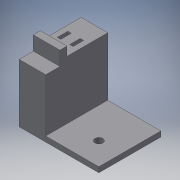
# Autodesk Inventor part: FixedFiber
Saved by Autodesk Inventor 2019 (Build 230136000, 136)
## iProperties
Created: 2019-06-10
Part Number: FixedFiber
Material: Generic
Document SubType Name: Modeling
Designer: aorfi
Density: 1 g/cm^3
Appearance: Default
Author: aorfi
Autodesk Inventor part; units mm, degrees
ref_plane "YZ Plane" through (0, 0, 0) normal (1, 0, 0) x (0, 1, 0)
ref_plane "XZ Plane" through (0, 0, 0) normal (0, 1, 0) x (-1, 0, 0)
ref_plane "XY Plane" through (0, 0, 0) normal (0, 0, 1) x (1, 0, 0)
sketch "Sketch1" plane through (0, 0, 0) normal (0, 1, 0) x (-1, 0, 0)
  line L0 (-22.5, 17.5) -> (22.5, 17.5)
  line L1 (22.5, 17.5) -> (22.5, -17.5)
  line L2 (22.5, -17.5) -> (-22.5, -17.5)
  line L3 (-22.5, -17.5) -> (-22.5, 17.5)
  line L4 (-22.5, 17.5) -> (22.5, -17.5) construction
  line L5 (22.5, 17.5) -> (-22.5, -17.5) construction
  point P0 (0, 0)
  dimension "d0" = 35
  dimension "d1" = 45
  constraints: 12 end point, 2 midpoint, 2 parallel, 1 horizontal, 1 perpendicular
  measures "d0" distance of L0.end L1.end
  measures "d1" distance of L1.end L2.end
extrude "Extrusion1" add sketch "Sketch1" along normal mid plane 3
sketch "Sketch2" plane through (0, 1.5, 0) normal (0, 1, 0) x (1, 0, 0)
  line L0 (-22.5, -17.5) -> (22.5, -17.5) projected
  line L1 (22.5, -17.5) -> (22.5, 17.5) projected
  point P0 (9.8, -4.8)
  dimension "d11" = 12.7
  dimension "d12" = 12.7
  measures "d11" distance from line of L0 point (9.8, -4.8)
  measures "d12" distance from line of L1 point (9.8, -4.8)
hole "Hole1" at (9.8, 1.5, 4.8) direction (0, -1, 0) diameter 4.496 end through all clearance for "Flat Head Machine Screw (82)" size "#8" standard "Ansi Unified Screw Threads"
sketch "Sketch3" plane through (0, 1.5, 0) normal (0, 1, 0) x (1, 0, 0)
  line L0 (22.5, 17.5) -> (-22.5, 17.5) projected
  line L1 (-22.5, 17.5) -> (-7.5, 17.5)
  line L2 (-7.5, 17.5) -> (-7.5, -17.5)
  line L3 (-7.5, -17.5) -> (-22.5, -17.5)
  line L4 (-22.5, -17.5) -> (-22.5, 17.5)
  line L5 (-22.5, -17.5) -> (22.5, -17.5) projected
  point P0 (0, 0)
  dimension "d13" = 15
  constraints: 8 end point, 2 parallel, 1 collinear, 1 horizontal, 1 perpendicular
  measures "d13" distance of L2.end L3.end
extrude "Extrusion2" add sketch "Sketch3" along normal blind 33
sketch "Sketch4" plane through (0, 34.5, 0) normal (0, 1, 0) x (1, 0, 0)
  line L0 (-7.5, -17.5) -> (-7.5, 17.5) projected
  line L1 (-22.5, -3.5) -> (-7.5, -3.5)
  line L2 (-7.5, -3.5) -> (-7.5, -7.5)
  line L3 (-7.5, -7.5) -> (-22.5, -7.5)
  line L4 (-22.5, -7.5) -> (-22.5, -3.5)
  line L5 (-22.5, 17.5) -> (-22.5, -17.5) projected
  line L6 (-22.5, -3.5) -> (-7.5, -3.5) construction
  line L7 (-7.5, -3.5) -> (-7.5, 3.5) construction
  line L8 (-7.5, 3.5) -> (-22.5, 3.5) construction
  line L9 (-22.5, 3.5) -> (-22.5, -3.5) construction
  line L10 (-22.5, -17.5) -> (-22.5, 17.5) construction
  line L11 (-22.5, 0) -> (-7.5, 0) construction
  line L12 (-22.5, -17.5) -> (-7.5, -17.5) projected
  point P0 (0, 0)
  dimension "d16" = 4
  dimension "d32" = 10
  constraints: 18 end point, 4 parallel, 4 point on line, 3 horizontal, 2 collinear, 2 midpoint, 2 perpendicular
  measures "d16" distance between parallel lines of L3 L1
  measures "d32" distance between parallel lines of L12 L3
extrude "Extrusion3" add sketch "Sketch4" along normal blind 5 contours L3 L4 L1 L0
sketch "Sketch5" plane through (0, 34.5, 0) normal (0, 1, 0) x (1, 0, 0)
  line L0 (-19.5, 9) -> (-17.5, 9)
  line L1 (-17.5, 9) -> (-17.5, 3)
  line L2 (-17.5, 3) -> (-19.5, 3)
  line L3 (-19.5, 3) -> (-19.5, 9)
  line L4 (-10.5, 9) -> (-12.5, 9)
  line L5 (-12.5, 9) -> (-12.5, 3)
  line L6 (-12.5, 3) -> (-10.5, 3)
  line L7 (-10.5, 3) -> (-10.5, 9)
  line L8 (-18.5, 6) -> (-11.5, 6) construction
  line L9 (-7.5, -3.5) -> (-22.5, -3.5) construction
  line L10 (-7.5, 11.5) -> (-7.5, 1.5) construction
  line L11 (-7.5, 1.5) -> (-22.5, 1.5) construction
  line L12 (-22.5, 17.5) -> (-22.5, -3.5) construction
  line L13 (-22.5, -17.5) -> (-22.5, 17.5) construction
  point P0 (0, 0)
  point P1 (-15, -3.5)
  point P2 (-15, 6)
  point P3 (-11.5, 9)
  point P4 (-18.5, 9)
  point P5 (-17.5, 6)
  dimension "d20" = 6
  dimension "d21" = 2
  dimension "d22" = 5
  dimension "d26" = 1.5
  dimension "d31" = 7
  constraints: 22 end point, 5 midpoint, 4 parallel, 3 horizontal, 3 point on line, 3 vertical alignment, 2 perpendicular, 1 collinear
  measures "d20" distance of L2.end L0.start
  measures "d21" distance of L0.start L0.end
  measures "d22" distance between parallel lines of L9 L11
  measures "d26" distance between parallel lines of L2 L11
  measures "d31" distance of L8.start L8.end
extrude "Extrusion4" cut sketch "Sketch5" against normal blind 3
sketch "Sketch7" plane through (-22.5, -1.5, -17.5) normal (-1, 0, 0) x (0, 0, 1)
  line L0 (35, 36) -> (25, 36)
  line L1 (25, 36) -> (25, 33)
  line L2 (25, 33) -> (35, 33)
  line L3 (35, 33) -> (35, 36)
  line L4 (25, 36) -> (25, 41) projected
  point P0 (17.5, 1.5)
  dimension "d33" = 3
  constraints: 8 end point, 2 parallel, 1 collinear, 1 horizontal, 1 perpendicular
  measures "d33" distance between parallel lines of L2 L0
extrude "Extrusion6" cut sketch "Sketch7" against normal through all
sketch "Sketch8" plane through (0, 34.5, 0) normal (0, 1, 0) x (1, 0, 0)
  line L0 (-22.5, -3.5) -> (-7.5, -3.5) projected
  line L1 (-7.5, -3.5) -> (-8.5, -3.5)
  line L2 (-8.5, -3.5) -> (-8.5, -1.5)
  line L3 (-8.5, -1.5) -> (-7.5, -1.5)
  line L4 (-7.5, -1.5) -> (-7.5, -3.5)
  point P0 (0, 0)
  dimension "d36" = 1
  dimension "d37" = 2
  constraints: 8 end point, 2 parallel, 1 horizontal, 1 perpendicular
  measures "d36" distance of L2.end L3.end
  measures "d37" distance of L1.end L2.end
extrude "Extrusion7" add sketch "Sketch8" along normal blind 1
body "Solid1"
